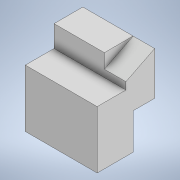
# Autodesk Inventor part: 4
Saved by Autodesk Inventor 2022 (Build 260153000, 153)
## iProperties
Created: 2022-03-14
Part Number: 4
Material: Všeobecné
Document SubType Name: Modeling
Designer: Šimon
Density: 1 g/cm^3
Appearance: Výchozí
Author: Šimon
Autodesk Inventor part; units mm, degrees
ref_plane "YZ Plane" through (0, 0, 0) normal (1, 0, 0) x (0, 1, 0)
ref_plane "XZ Plane" through (0, 0, 0) normal (0, 1, 0) x (-1, 0, 0)
ref_plane "XY Plane" through (0, 0, 0) normal (0, 0, 1) x (1, 0, 0)
sketch "Náčrt1" plane through (0, 0, 0) normal (1, 0, 0) x (0, 1, 0)
  line L0 (0, 0) -> (0, -25)
  line L1 (0, -25) -> (25, -25)
  line L2 (25, -25) -> (25, -40)
  line L3 (25, -40) -> (55, -40)
  line L4 (55, -40) -> (55, -20)
  line L5 (55, -20) -> (40, -20)
  line L6 (40, -20) -> (40, 0)
  line L7 (40, 0) -> (0, 0)
  dimension "d0" = 25
  dimension "d1" = 25
  dimension "d2" = 15
  dimension "d3" = 30
  dimension "d4" = 20
  dimension "d5" = 15
  dimension "d6" = 20
  constraints: 16 end point, 6 perpendicular, 1 vertical
  measures "d0" distance of L0.start L0.end
  measures "d1" distance of L0.end L1.end
  measures "d2" distance of L1.end L2.end
  measures "d3" distance of L2.end L3.end
  measures "d4" distance of L3.end L4.end
  measures "d5" distance of L4.end L5.end
  measures "d6" distance of L5.end L6.end
extrude "Vysunutí1" add sketch "Náčrt1" along normal blind 50
sketch "Náčrt2" plane through (50, 0, 0) normal (1, 0, 0) x (0, 0, -1)
  line L0 (20, 55) -> (20, 40) projected
  line L1 (40, 55) -> (20, 55) projected
  line L2 (20, 45) -> (40, 55)
  line L3 (40, 25) -> (40, 55) projected
  line L4 (40, 55) -> (20, 55)
  point P0 (0, 0)
  constraints: 4 end point, 1 horizontal, 1 point on line
extrude "Vysunutí2" cut sketch "Náčrt2" against normal blind 15
